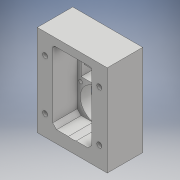
# Autodesk Inventor part: servotestarm90back
Saved by Autodesk Inventor 2018 (Build 220112000, 112)
## iProperties
Created: 2018-02-01
Part Number: servotestarm90back
Material: Generic
Document SubType Name: Modeling
Designer: Clevo
Density: 1 g/cm^3
Appearance: Default
Author: Clevo
Autodesk Inventor part; units mm, degrees
ref_plane "YZ Plane" through (0, 0, 0) normal (1, 0, 0) x (0, 1, 0)
ref_plane "XZ Plane" through (0, 0, 0) normal (0, 1, 0) x (-1, 0, 0)
ref_plane "XY Plane" through (0, 0, 0) normal (0, 0, 1) x (1, 0, 0)
sketch "Sketch1" plane through (0, 0, 0) normal (0, 1, 0) x (-1, 0, 0)
  line L0 (12.25, 22.5) -> (-12.25, 22.5)
  line L1 (-12.25, 22.5) -> (-12.25, -22.5)
  line L2 (-12.25, -22.5) -> (12.25, -22.5)
  line L3 (12.25, -22.5) -> (12.25, 22.5)
  point P0 (0, 0)
  point P1 (12.25, 0)
  point P2 (0, 22.5)
  dimension "d0" = 24.5
  dimension "d1" = 45
  constraints: 8 end point, 2 midpoint, 2 parallel, 1 horizontal, 1 horizontal alignment, 1 perpendicular, 1 vertical alignment
  measures "d0" distance of L2.end L1.end
  measures "d1" distance of L1.end L0.end
extrude "Extrusion1" add sketch "Sketch1" along normal blind 1.95
sketch "Sketch2" plane through (0, 1.95, 0) normal (0, 1, 0) x (1, 0, 0)
  line L0 (-10, 1.25) -> (10, 1.25)
  line L1 (10, 1.25) -> (10, -17.25)
  line L2 (10, -17.25) -> (-10, -17.25)
  line L3 (-10, -17.25) -> (-10, 1.25)
  line L4 (-12.25, -22.5) -> (12.25, -22.5) projected
  line L5 (12.25, -22.5) -> (12.25, 22.5) projected
  line L6 (12.25, 22.5) -> (-12.25, 22.5) projected
  line L7 (-12.25, 22.5) -> (-12.25, -22.5) projected
  line L8 (-7, -17.25) -> (7, -17.25)
  line L9 (7, -17.25) -> (7, -22.5)
  line L10 (7, -22.5) -> (-7, -22.5)
  line L11 (-7, -22.5) -> (-7, -17.25)
  line L12 (-12.25, -22.5) -> (12.25, -22.5) projected
  point P0 (0, 0)
  dimension "d4" = 2.25
  dimension "d5" = 20
  dimension "d6" = 2.25
  dimension "d7" = 5.25
  dimension "d8" = 5.25
  dimension "d9" = 14
  dimension "d10" = 5.25
  dimension "d11" = 18.5
  constraints: 16 end point, 4 parallel, 2 horizontal, 2 perpendicular, 1 collinear, 1 point on line
  measures "d4" distance between parallel lines of L7 L3
  measures "d5" distance of L0.start L0.end
  measures "d6" distance between parallel lines of L5 L1
  measures "d7" distance of L8.end L9.end
  measures "d8" distance between parallel lines of L7 L11
  measures "d9" distance between parallel lines of L9 L11
  measures "d10" distance between parallel lines of L5 L9
  measures "d11" distance of L0.end L1.end
extrude "Extrusion2" cut sketch "Sketch2" against normal up to surface (1.95 mm away) contours L0 L1 L2 L3 | L2 L9 L4 L11
sketch "Sketch3" plane through (0, 1.95, 0) normal (0, 1, 0) x (1, 0, 0)
  line L0 (-7, -22.5) -> (-7, -17.25) projected
  line L1 (-7, -17.25) -> (-10, -17.25) projected
  line L2 (-10, -17.25) -> (-10, 1.25) projected
  line L3 (-10, 1.25) -> (10, 1.25) projected
  line L4 (10, 1.25) -> (10, -17.25) projected
  line L5 (10, -17.25) -> (7, -17.25) projected
  line L6 (7, -17.25) -> (7, -22.5) projected
  line L7 (7, -22.5) -> (12.25, -22.5) projected
  line L8 (12.25, -22.5) -> (12.25, 22.5) projected
  line L9 (12.25, 22.5) -> (-12.25, 22.5) projected
  line L10 (-12.25, 22.5) -> (-12.25, -22.5) projected
  line L11 (-12.25, -22.5) -> (-7, -22.5) projected
  point P0 (0, 0)
  point P1 (-10.25, -20.305)
  point P2 (10.25, -20.305)
  dimension "d14" = 20.5
  dimension "d15" = 2
  dimension "d16" = 2.195
  dimension "d17" = 2
  constraints: 1 horizontal alignment
  measures "d14" distance of point (10.25, -20.305) point (-10.25, -20.305)
  measures "d15" distance from line of L8 point (10.25, -20.305)
  measures "d16" distance from line of L11 point (-10.25, -20.305)
  measures "d17" distance from line of L10 point (-10.25, -20.305)
hole "Hole1" at (-10.25, 1.95, 20.305) at (10.25, 1.95, 20.305) direction (0, -1, 0) diameter 2.4 end through all clearance for "Flat Head Machine Screw" size "M2" standard "Ansi Metric M Profile"
sketch "Sketch4" plane through (0, 1.95, 0) normal (0, 1, 0) x (1, 0, 0)
  circle A0 centre (-10.25, -20.305) radius 1.2 projected
  circle A1 centre (10.25, -20.305) radius 1.2 projected
  line L0 (-7, -22.5) -> (-7, -17.25) projected
  line L1 (-7, -17.25) -> (-10, -17.25) projected
  line L2 (-10, -17.25) -> (-10, 1.25) projected
  line L3 (-10, 1.25) -> (10, 1.25) projected
  line L4 (10, 1.25) -> (10, -17.25) projected
  line L5 (10, -17.25) -> (7, -17.25) projected
  line L6 (7, -17.25) -> (7, -22.5) projected
  line L7 (7, -22.5) -> (12.25, -22.5) projected
  line L8 (12.25, -22.5) -> (12.25, 22.5) projected
  line L9 (12.25, 22.5) -> (-12.25, 22.5) projected
  line L10 (-12.25, 22.5) -> (-12.25, -22.5) projected
  line L11 (-12.25, -22.5) -> (-7, -22.5) projected
  point P0 (0, 0)
  point P1 (-10.25, 4.15)
  point P2 (10.25, 4.15)
  dimension "d25" = 20.5
  dimension "d26" = 26.65
  dimension "d27" = 2
  dimension "d28" = 2
  constraints: 1 horizontal alignment
  measures "d25" distance of point (10.25, 4.15) point (-10.25, 4.15)
  measures "d26" distance from line of L11 point (-10.25, 4.15)
  measures "d27" distance from line of L10 point (-10.25, 4.15)
  measures "d28" distance from line of L8 point (10.25, 4.15)
hole "Hole2" at (-10.25, 1.95, -4.15) at (10.25, 1.95, -4.15) direction (0, -1, 0) diameter 2.4 end through all clearance for "Flat Head Machine Screw" size "M2" standard "Ansi Metric M Profile"
fillet "Fillet1" radius 0.5 2 edges at (7, 0.975, 17.25) (-7, 0.975, 17.25)
sketch "Sketch5" plane through (0, 1.95, 0) normal (0, 1, 0) x (1, 0, 0)
  circle A0 centre (-10.25, 4.15) radius 1.2 projected
  circle A1 centre (10.25, 4.15) radius 1.2 projected
  circle A2 centre (-10.25, -20.305) radius 1.2 projected
  circle A3 centre (10.25, -20.305) radius 1.2 projected
  arc A4 (-7, -17.75) -> (-7.5, -17.25) centre (-7.5, -17.75) ccw projected
  line L0 (-7.5, -17.25) -> (-10, -17.25) projected
  line L1 (-10, -17.25) -> (-10, 1.25) projected
  line L2 (-10, 1.25) -> (10, 1.25) projected
  line L3 (10, 1.25) -> (10, -17.25) projected
  line L4 (10, -17.25) -> (7.5, -17.25) projected
  arc A5 (7.5, -17.25) -> (7, -17.75) centre (7.5, -17.75) ccw projected
  line L5 (7, -17.75) -> (7, -22.5) projected
  line L6 (7, -22.5) -> (12.25, -22.5) projected
  line L7 (12.25, -22.5) -> (12.25, 22.5) projected
  line L8 (12.25, 22.5) -> (-12.25, 22.5) projected
  line L9 (-12.25, 22.5) -> (-12.25, -22.5) projected
  line L10 (-12.25, -22.5) -> (-7, -22.5) projected
  line L11 (-7, -22.5) -> (-7, -17.75) projected
  line L12 (-12.25, 22.5) -> (-12.25, -22.5) projected
  line L13 (12.25, -22.5) -> (12.25, 22.5) projected
  line L14 (-12.25, -22.5) -> (12.25, -22.5)
  line L15 (12.25, -22.5) -> (12.25, -4.5)
  line L16 (12.25, -4.5) -> (10, -4.5)
  line L17 (-12.25, -4.5) -> (-12.25, -22.5)
  line L18 (-10, -4.5) -> (-12.25, -4.5)
  line L19 (10, -4.5) -> (-10, -4.5)
  point P0 (0, 0)
  dimension "d37" = 18
  constraints: 12 end point, 4 parallel, 3 point on line, 1 horizontal, 1 perpendicular
  measures "d37" distance between parallel lines of L14 L16
extrude "Extrusion3" add sketch "Sketch5" along normal blind 5 contours L11 L10 L9 L18 L1 L0 A4 | A4 L0 L1 L19 L3 L4 A5 L5 L14 L11 | L5 A5 L4 L3 L16 L7 L6 | L18 L9 L8 L7 L16 L3 L2 L1
sketch "Sketch6" plane through (12.25, 0, 22.5) normal (1, 0, 0) x (0, 0, -1)
  line L0 (0, 0) -> (45, 0) projected
  line L1 (45, 0) -> (45, 6.95) projected
  line L2 (0, 6.95) -> (45, 6.95) projected
  line L3 (0, 0) -> (0, 6.95) projected
  line L4 (45, 0) -> (45, 6.95) projected
  line L5 (45, 6.95) -> (0, 6.95)
  line L6 (0, 6.95) -> (0, -32)
  line L7 (0, -32) -> (45, -32)
  line L8 (45, -32) -> (45, 6.95)
  line L9 (0, 0) -> (0, 6.95) projected
  line L10 (0, 0) -> (45, 0) projected
  line L11 (45, 0) -> (0, 0)
  line L12 (0, 0) -> (0, -32)
  line L13 (0, -32) -> (45, -32)
  line L14 (45, -32) -> (45, 0)
  point P0 (22.5, 0)
  dimension "d72" = 32
  constraints: 16 end point, 4 parallel, 2 horizontal, 2 perpendicular, 1 collinear
  measures "d72" distance between parallel lines of L0 L7
extrude "Extrusion4" add sketch "Sketch6" along normal blind 10
sketch "Sketch7" plane through (12.25, -32, -22.5) normal (0, -1, 0) x (1, 0, 0)
  line L0 (0, 45) -> (0, 0) projected
  line L1 (0, 0) -> (10, 0) projected
  line L2 (10, 45) -> (10, 0) projected
  line L3 (0, 45) -> (10, 45) projected
  line L4 (0, 0) -> (-24.5, 0) projected
  line L5 (0, 0) -> (-24.5, 0)
  line L6 (-24.5, 0) -> (-24.5, 45)
  line L7 (-24.5, 45) -> (0, 45)
  line L8 (0, 45) -> (0, 0)
  point P0 (-12.25, 22.5)
  dimension "d43" = 24.5
  constraints: 8 end point, 2 parallel, 1 collinear, 1 horizontal, 1 perpendicular
  measures "d43" distance of L0.end L5.end
extrude "Extrusion5" add sketch "Sketch7" along normal blind 1.15
sketch "Sketch8" plane through (12.25, -33.15, -22.5) normal (0, -1, 0) x (1, 0, 0)
  line L0 (-24.5, 0) -> (10, 0) projected
  line L1 (10, 0) -> (10, 45) projected
  line L2 (10, 45) -> (-24.5, 45) projected
  line L3 (-24.5, 45) -> (-24.5, 0) projected
  circle A0 centre (-12.25, 10) radius 10.5
  line L4 (-19.25, 45) -> (-5.25, 45) projected
  line L5 (-5, 45) -> (-19.5, 45)
  line L6 (-19.5, 45) -> (-19.5, 36)
  line L7 (-19.5, 36) -> (-5, 36)
  line L8 (-5, 36) -> (-5, 45)
  line L9 (-2.25, 21.25) -> (-22.25, 21.25)
  line L10 (-22.25, 21.25) -> (-22.25, 36)
  line L11 (-22.25, 36) -> (-2.25, 36)
  line L12 (-2.25, 36) -> (-2.25, 21.25)
  line L13 (-5, 21.25) -> (-19.5, 21.25)
  line L14 (-19.5, 21.25) -> (-19.5, 17.25)
  line L15 (-19.5, 17.25) -> (-5, 17.25)
  line L16 (-5, 17.25) -> (-5, 21.25)
  line L17 (-24.5, 0) -> (10, 0) projected
  line L18 (-24.5, 45) -> (0, 45)
  line L19 (0, 45) -> (0, 0)
  line L20 (0, 0) -> (-24.5, 0)
  line L21 (-24.5, 0) -> (-24.5, 45)
  point P0 (-12.25, 22.5)
  dimension "d46" = 10
  dimension "d47" = 21
  dimension "d48" = 14.5
  dimension "d49" = 20
  dimension "d50" = 14.5
  dimension "d51" = 24.5
  dimension "d52" = 5
  dimension "d53" = 5
  dimension "d54" = 2.25
  dimension "d55" = 2.25
  dimension "d56" = 5
  dimension "d57" = 5
  dimension "d58" = 9
  dimension "d59" = 14.75
  dimension "d60" = 4
  constraints: 32 end point, 8 parallel, 4 horizontal, 4 perpendicular, 4 point on line, 1 centre point, 1 vertical alignment
  measures "d46" distance from line of L0 A0.centre
  measures "d47" diameter of A0
  measures "d48" distance between parallel lines of L6 L8
  measures "d49" distance of L10.end L11.end
  measures "d50" distance of L14.end L15.end
  measures "d51" distance between parallel lines of L3 L19
  measures "d52" distance between parallel lines of L19 L16
  measures "d53" distance between parallel lines of L3 L14
  measures "d54" distance between parallel lines of L19 L12
  measures "d55" distance between parallel lines of L3 L10
  measures "d56" distance between parallel lines of L3 L6
  measures "d57" distance between parallel lines of L19 L8
  measures "d58" distance of L5.end L6.end
  measures "d59" distance of L9.end L10.end
  measures "d60" distance of L13.end L14.end
extrude "Extrusion6" cut sketch "Sketch8" against normal up to surface (1.15 mm away) contours A0 L0 | L0 A0 L14 L15 L16 | L8 L7 L6 L2 | L14 L9 L16 A0 | A0 L16 L15 L14 | L11 L12 L9 L10 L7
sketch "Sketch9" plane through (12.25, -33.15, -22.5) normal (0, -1, 0) x (1, 0, 0)
  line L0 (-5, 45) -> (-5, 36) projected
  line L1 (-5, 36) -> (-2.25, 36) projected
  line L2 (-2.25, 36) -> (-2.25, 21.25) projected
  line L3 (-2.25, 21.25) -> (-5, 21.25) projected
  line L4 (-5, 21.25) -> (-5, 17.5952) projected
  arc A0 (-9.0484, 0) -> (-5, 17.5952) centre (-12.25, 10) ccw projected
  line L5 (-9.0484, 0) -> (10, 0) projected
  line L6 (10, 0) -> (10, 45) projected
  line L7 (10, 45) -> (-5, 45) projected
  line L8 (-19.5, 36) -> (-19.5, 45) projected
  line L9 (-19.5, 45) -> (-24.5, 45) projected
  line L10 (-24.5, 45) -> (-24.5, 0) projected
  line L11 (-24.5, 0) -> (-15.4516, 0) projected
  arc A1 (-19.5, 17.5952) -> (-15.4516, 0) centre (-12.25, 10) ccw projected
  line L12 (-19.5, 17.5952) -> (-19.5, 21.25) projected
  line L13 (-19.5, 21.25) -> (-22.25, 21.25) projected
  line L14 (-22.25, 21.25) -> (-22.25, 36) projected
  line L15 (-22.25, 36) -> (-19.5, 36) projected
  circle A2 centre (-22.5, 18.35) radius 1.2 projected
  circle A3 centre (-2, 18.35) radius 1.2 projected
  circle A4 centre (-2, 42.805) radius 1.2 projected
  circle A5 centre (-22.5, 42.805) radius 1.2 projected
  line L16 (-2, 18.35) -> (-22.5, 18.35)
  line L17 (-22.5, 18.35) -> (-22.5, 39.05)
  line L18 (-22.5, 39.05) -> (-2, 39.05)
  line L19 (-2, 39.05) -> (-2, 18.35)
  point P0 (-12.25, 22.5)
  dimension "d63" = 20.7
  constraints: 8 end point, 2 parallel, 1 horizontal, 1 perpendicular, 1 point on line
  measures "d63" distance of L16.end L17.end
hole "Hole3" at (-10.25, -33.15, -4.15) at (10.25, -33.15, -4.15) at (10.25, -33.15, 16.55) at (-10.25, -33.15, 16.55) direction (0, 1, 0) diameter 2.4 depth 8 tip angle 118 clearance for "Flat Head Machine Screw" size "M2" standard "Ansi Metric M Profile"
sketch "Sketch10" plane through (12.25, -33.15, -22.5) normal (0, -1, 0) x (1, 0, 0)
  circle A0 centre (-2, 39.05) radius 1.2 projected
  circle A1 centre (-2, 18.35) radius 1.2 projected
  line L0 (-5, 45) -> (-5, 36) projected
  line L1 (-5, 36) -> (-2.25, 36) projected
  line L2 (-2.25, 36) -> (-2.25, 21.25) projected
  line L3 (-2.25, 21.25) -> (-5, 21.25) projected
  line L4 (-5, 21.25) -> (-5, 17.5952) projected
  arc A2 (-9.0484, 0) -> (-5, 17.5952) centre (-12.25, 10) ccw projected
  line L5 (-9.0484, 0) -> (10, 0) projected
  line L6 (10, 0) -> (10, 45) projected
  line L7 (10, 45) -> (-5, 45) projected
  circle A3 centre (-22.5, 18.35) radius 1.2 projected
  circle A4 centre (-22.5, 39.05) radius 1.2 projected
  line L8 (-19.5, 36) -> (-19.5, 45) projected
  line L9 (-19.5, 45) -> (-24.5, 45) projected
  line L10 (-24.5, 45) -> (-24.5, 0) projected
  line L11 (-24.5, 0) -> (-15.4516, 0) projected
  arc A5 (-19.5, 17.5952) -> (-15.4516, 0) centre (-12.25, 10) ccw projected
  line L12 (-19.5, 17.5952) -> (-19.5, 21.25) projected
  line L13 (-19.5, 21.25) -> (-22.25, 21.25) projected
  line L14 (-22.25, 21.25) -> (-22.25, 36) projected
  line L15 (-22.25, 36) -> (-19.5, 36) projected
  line L16 (10, 0) -> (10, 45) projected
  line L17 (-24.5, 0) -> (-24.5, 45) projected
  line L18 (10, 0) -> (-24.5, 0)
  line L19 (-24.5, 0) -> (-24.5, 45)
  line L20 (-24.5, 45) -> (10, 45)
  line L21 (10, 45) -> (10, 0)
  arc A6 (-19.5, 17.5952) -> (-15.4516, 0) centre (-12.25, 10) ccw projected
  circle A7 centre (-12.25, 10) radius 10.5
  point P0 (-12.25, 22.5)
  constraints: 8 end point, 2 parallel, 1 coincident, 1 horizontal, 1 perpendicular, 3 other
extrude "Extrusion7" add sketch "Sketch10" along normal blind 5
sketch "Sketch11" plane through (12.25, -38.15, -22.5) normal (0, -1, 0) x (1, 0, 0)
  line L0 (-9.0484, 0) -> (10, 0) projected
  line L1 (10, 0) -> (10, 45) projected
  line L2 (10, 45) -> (-24.5, 45) projected
  line L3 (-24.5, 45) -> (-24.5, 0) projected
  line L4 (-24.5, 0) -> (-15.4516, 0) projected
  arc A0 (-15.4516, 0) -> (-9.0484, 0) centre (-12.25, 10) ccw projected
  arc A1 (-19.5, 17.5952) -> (-15.4516, 0) centre (-12.25, 10) ccw projected
  circle A2 centre (-12.25, 10) radius 10.5
  point P0 (-12.25, 22.5)
  constraints: 1 coincident, 3 other
extrude "Extrusion8" cut sketch "Sketch11" against normal up to surface (5 mm away) contours A0 A1 A2
sketch "Sketch12" plane through (-12.25, 0, -22.5) normal (-1, 0, 0) x (0, 0, 1)
  line L0 (-6.0754, -39.5109) -> (50.3226, -39.5109)
  line L1 (50.3226, -39.5109) -> (50.3226, 16.733)
  line L2 (50.3226, 16.733) -> (-6.0754, 16.733)
  line L3 (-6.0754, 16.733) -> (-6.0754, -39.5109)
  point P0 (22.5, 0)
  constraints: 8 end point, 2 parallel, 1 horizontal, 1 perpendicular
extrude "Extrusion9" cut sketch "Sketch12" against normal blind 12.25
sketch "Sketch13" plane through (0, 0, 0) normal (0, -1, 0) x (1, 0, 0)
  arc A0 (3.2016, -22.5) -> (0, -2) centre (0, -12.5) ccw projected
  circle A1 centre (0, -12.5) radius 4
  point P0 (0, 0)
  dimension "d80" = 8
  constraints: 1 centre point, 1 coincident
  measures "d80" diameter of A1
extrude "Extrusion10" cut sketch "Sketch13" against normal blind 4.5
sketch "Sketch14" plane through (12.25, 0, 22.5) normal (-1, 0, 0) x (0, 0, 1)
  line L0 (0, 0) -> (-45, 0) projected
  line L1 (-45, -32) -> (-45, 0) projected
  line L2 (0, -32) -> (-45, -32) projected
  line L3 (0, 0) -> (0, -32) projected
  point P0 (-22.5, 0)
extrude "Extrusion11" cut sketch "Sketch14" against normal blind 0.2
sketch "Sketch15" plane through (0, 6.95, 0) normal (0, 1, 0) x (1, 0, 0)
  arc A0 (0, 8.5) -> (0, 16.5) centre (0, 12.5) ccw projected
  circle A1 centre (0, 12.5) radius 10.5
  point P0 (0, 0)
  dimension "d86" = 21
  constraints: 1 centre point, 1 coincident
  measures "d86" diameter of A1
extrude "Extrusion12" cut sketch "Sketch15" against normal up to surface (6.95 mm away)
sketch "Sketch16" plane through (22.25, -38.15, -22.5) normal (0, 0, -1) x (-1, 0, 0)
  line L0 (19.0484, 45.1) -> (0, 45.1) projected
  line L1 (0, 45.1) -> (0, 0) projected
  line L2 (19.0484, 0) -> (0, 0) projected
  line L3 (19.0484, 6.15) -> (9.8, 6.15) projected
  line L4 (9.8, 6.15) -> (9.8, 38.15) projected
  line L5 (9.8, 38.15) -> (19.0484, 38.15) projected
  line L6 (22.25, 45.1) -> (22.25, 40.1) projected
  line L7 (0, 0) -> (22.25, 0)
  line L8 (22.25, 0) -> (22.25, 45.1)
  line L9 (22.25, 45.1) -> (0, 45.1)
  line L10 (0, 45.1) -> (0, 0)
  line L11 (19.0484, 38.15) -> (19.0484, 45.1) projected
  line L12 (19.0484, 0) -> (19.0484, 6.15) projected
  point P0 (22.25, 38.15)
  constraints: 8 end point, 2 parallel, 1 horizontal, 1 perpendicular
extrude "Extrusion13" add sketch "Sketch16" along normal blind 8
sketch "Sketch17" plane through (7, 0, 22.5) normal (0, 0, 1) x (1, 0, 0)
  line L0 (0, 0) -> (5.45, 0) projected
  line L1 (5.45, 0) -> (5.45, -32) projected
  line L2 (5.45, -32) -> (0.25, -32) projected
  line L3 (0.25, -32) -> (0.25, -33.15) projected
  line L4 (0.25, -33.15) -> (-7, -33.15) projected
  line L5 (-7, -33.15) -> (-7, -38.15) projected
  line L6 (15.25, -38.15) -> (-7, -38.15) projected
  line L7 (15.25, 6.95) -> (15.25, -38.15) projected
  line L8 (-7, 6.95) -> (15.25, 6.95) projected
  line L9 (-7, 6.95) -> (-7, 1.95) projected
  line L10 (-7, 1.95) -> (0, 1.95) projected
  line L11 (0, 1.95) -> (0, 0) projected
  line L12 (-7, 6.95) -> (15.25, 6.95) projected
  line L13 (-7, -38.15) -> (-7, -33.15) projected
  line L14 (15.25, 6.95) -> (-7, 6.95)
  line L15 (-7, 6.95) -> (-7, -38.15)
  line L16 (-7, -38.15) -> (15.25, -38.15)
  line L17 (15.25, -38.15) -> (15.25, 6.95)
  point P0 (-7, 0)
  constraints: 8 end point, 2 parallel, 1 horizontal, 1 perpendicular
extrude "Extrusion14" add sketch "Sketch17" along normal blind 5
sketch "Sketch18" plane through (12.25, -38.15, -22.5) normal (0, -1, 0) x (1, 0, 0)
  line L0 (-12.25, 50) -> (-12.25, 20.5) projected
  arc A0 (-9.0484, 0) -> (-12.25, 20.5) centre (-12.25, 10) ccw projected
  line L1 (-9.0484, 0) -> (-12.25, 0) projected
  line L2 (-12.25, 0) -> (-12.25, -8) projected
  line L3 (10, -8) -> (-12.25, -8) projected
  line L4 (10, 50) -> (10, -8) projected
  line L5 (-12.25, 50) -> (10, 50) projected
  circle A1 centre (-2, 39.05) radius 1.2 projected
  circle A2 centre (-2, 18.35) radius 1.2 projected
  line L6 (-12.25, 21.25) -> (-12.25, 20.5) projected
  circle A3 centre (-12.25, 10) radius 10.5
  point P0 (-12.25, 22.5)
  constraints: 1 coincident, 1 vertical alignment, 2 other
extrude "Extrusion15" cut sketch "Sketch18" against normal up to surface (45.1 mm away) contours A0 L1 L2 A3 | L2 L1 A3
sketch "Sketch19" plane through (22.25, -38.15, -22.5) normal (0, 0, 1) x (1, 0, 0)
  line L0 (-19.0484, 38.15) -> (-19.0484, 6.15) projected
  line L1 (-19.0484, 6.15) -> (-9.8, 6.15) projected
  line L2 (-9.8, 6.15) -> (-9.8, 38.15) projected
  line L3 (-9.8, 38.15) -> (-19.0484, 38.15) projected
  line L4 (-9.8, 38.15) -> (-39.7398, 38.15)
  line L5 (-39.7398, 38.15) -> (-39.7398, 6.15)
  line L6 (-39.7398, 6.15) -> (-9.8, 6.15)
  line L7 (-9.8, 6.15) -> (-9.8, 38.15)
  point P0 (-22.25, 38.15)
  constraints: 8 end point, 2 parallel, 1 collinear, 1 horizontal, 1 perpendicular
extrude "Extrusion16" cut sketch "Sketch19" against normal blind 0.2
sketch "Sketch20" plane through (7, 0, 22.5) normal (0, 0, -1) x (-1, 0, 0)
  line L0 (-0.25, -33.15) -> (7, -33.15) projected
  line L1 (7, 1.95) -> (7, -33.15) projected
  line L2 (7, 1.95) -> (0, 1.95) projected
  line L3 (0, 1.95) -> (0, 0) projected
  line L4 (0, 0) -> (-5.45, 0) projected
  line L5 (-5.45, 0) -> (-5.45, -32) projected
  line L6 (-5.45, -32) -> (-0.25, -32) projected
  line L7 (-0.25, -32) -> (-0.25, -33.15) projected
  point P0 (7, 0)
extrude "Extrusion17" cut sketch "Sketch20" against normal blind 0.2
chamfer "Chamfer1" distance 2.5 angle 45 1 edges at (12.45, -16, -22.7)
fillet "Fillet7" radius 1.5 1 edges at (12.45, -16, 22.7)
fillet "Fillet8" radius 0.5 2 edges at (7.25, -32.575, -1.25) (7.25, -32.575, 13.5)
mirror "Mirror1" about plane through (0, -11.389, -0.3764) normal (-1, 0, 0)
sketch "Sketch22" plane through (0, 6.95, 0) normal (0, 1, 0) x (1, 0, 0)
  line L0 (-26.6142, 37.0922) -> (34.1584, 37.0922)
  line L1 (34.1584, 37.0922) -> (34.1584, -35.8349)
  line L2 (34.1584, -35.8349) -> (-26.6142, -35.8349)
  line L3 (-26.6142, -35.8349) -> (-26.6142, 37.0922)
  point P0 (0, 0)
  constraints: 8 end point, 2 parallel, 1 horizontal, 1 perpendicular
extrude "Extrusion18" cut sketch "Sketch22" against normal blind 22.55 keep common part
sketch "Sketch24" plane through (0, 0, 0) normal (0, -1, 0) x (1, 0, 0)
  line L0 (-17.25, 14.5) -> (17.25, 14.5)
  line L1 (17.25, 14.5) -> (17.25, -17.5)
  line L2 (17.25, -17.5) -> (-17.25, -17.5)
  line L3 (-17.25, -17.5) -> (-17.25, 14.5)
  line L4 (-10, -1.25) -> (10, -1.25) projected
  line L5 (10, -1.25) -> (10, 4.5) projected
  line L6 (-10, 4.5) -> (10, 4.5) projected
  line L7 (-10, -1.25) -> (-10, 4.5) projected
  circle A0 centre (0, -12.5) radius 10.5 projected
  circle A1 centre (-10.25, 20.305) radius 1.2 projected
  circle A2 centre (-10.25, -4.15) radius 1.2 projected
  line L8 (22.25, -30.5) -> (-22.25, -30.5) projected
  line L9 (-22.25, 27.5) -> (-22.25, -30.5) projected
  line L10 (22.25, 27.5) -> (-22.25, 27.5) projected
  line L11 (22.25, 27.5) -> (22.25, -30.5) projected
  circle A3 centre (10.25, -4.15) radius 1.2 projected
  circle A4 centre (10.25, 20.305) radius 1.2 projected
  point P0 (0, 0)
  dimension "d117" = 5
  dimension "d118" = 5
  dimension "d119" = 13
  dimension "d120" = 13
  constraints: 8 end point, 2 parallel, 1 horizontal, 1 perpendicular
  measures "d117" distance between parallel lines of L9 L3
  measures "d118" distance between parallel lines of L11 L1
  measures "d119" distance between parallel lines of L10 L0
  measures "d120" distance between parallel lines of L8 L2
hole "Hole5" at (-17.25, 0, -17.5) at (-17.25, 0, 14.5) at (17.25, 0, 14.5) at (17.25, 0, -17.5) direction (0, 1, 0) diameter 3.2 end through all both
equation "\"d4\" = d6"
equation "\"d8\" = d10"
equation "\"d15\" = d17"
equation "\"d27\" = d28"
equation "\"d52\" = d53"
equation "\"d54\" = d55"
equation "\"d56\" = d57"
equation "\"d118\" = d117"
body "Solid1"
